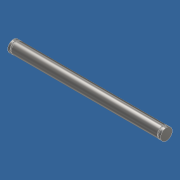
# Autodesk Inventor part: AxeHorizontalRoller
Saved by Autodesk Inventor 2018 (Build 220112000, 112)
## iProperties
Created: 2022-02-22
Part Number: AxeHorizontalRoller
Material: Stainless Steel
Document SubType Name: Modeling
Designer: Nathann
Density: 8 g/cm^3
Appearance: Semi-Polished
Mass: 40.2279 g
Surface Area: 30.1308 cm^2
Volume: 5.02849 cm^3
Author: Nathann
Autodesk Inventor part; units mm, degrees
ref_plane "YZ Plane" through (0, 0, 0) normal (1, 0, 0) x (0, 1, 0)
ref_plane "XZ Plane" through (0, 0, 0) normal (0, 1, 0) x (-1, 0, 0)
sketch "Sketch1" plane through (0, 0, 0) normal (1, 0, 0) x (0, 1, 0)
  arc A0 (-0.9778, 3.8786) -> (1.0222, 3.8672) centre (0, 0) ccw
  circle A1 centre (0, 0) radius 4
  dimension "d0" = 8
  constraints: 2 coincident, 2 point on circle, 1 centre point, 3 other
  measures "d0" diameter of A0
extrude "Extrusion1" add sketch "Sketch1" against normal blind 105
sketch "Sketch2" plane through (0, 0, 0) normal (0, 0, 1) x (1, 0, 0)
  line L0 (-2.44, 6.5) -> (-1.5, 6.5)
  line L1 (-1.5, 6.5) -> (-1.5, 3.5)
  line L2 (-1.5, 3.5) -> (-2.44, 3.5)
  line L3 (-2.44, 3.5) -> (-2.44, 6.5)
  line L4 (0, 4) -> (0, -4) projected
  line L5 (0, 4) -> (-105, 4) projected
  line L6 (-126, 0) -> (21, 0) projected
  line L7 (0, 4) -> (-105, 4) projected
  line L8 (-52.5, 4) -> (-52.5, -9.5088)
  line L9 (-102.56, 6.5) -> (-103.5, 6.5)
  line L10 (-103.5, 6.5) -> (-103.5, 3.5)
  line L11 (-103.5, 3.5) -> (-102.56, 3.5)
  line L12 (-102.56, 3.5) -> (-102.56, 6.5)
  line L13 (-105, 4) -> (-105, -4)
  line L14 (0, -4) -> (-105, -4) projected
  point P0 (0, 0)
  point P1 (0, 1.0222)
  point P2 (0, -0.9778)
  point P3 (-105, 0)
  point P4 (-105, 1.0222)
  point P5 (-105, -0.9778)
  dimension "d9" = 1.5
  dimension "d10" = 0.94
  dimension "d11" = 0.5
  dimension "d12" = 3
  dimension "d18" = 8
  constraints: 20 end point, 11 symmetric about line, 2 parallel, 1 horizontal, 1 midpoint, 1 perpendicular, 1 vertical
  measures "d9" distance between parallel lines of L4 L1
  measures "d10" distance of L1.end L2.end
  measures "d11" distance between parallel lines of L5 L2
  measures "d12" distance of L2.end L0.start
  measures "d18" distance between parallel lines of L5 L14
revolve "Revolution1" cut sketch "Sketch2" angle 360 about axis through (-10, 0, 0) along (1, 0, 0) contours L0 L1 L5 L3 | L5 L1 L2 L3 | L12 L11 L10 L5 | L5 L10 L9 L12
ref_plane "Work Plane1" through (0, 0, -4) normal (0, 0, 1) x (1, 0, 0)
sketch "Sketch5" plane through (0, 0, -4) normal (0, 0, 1) x (1, 0, 0)
  line L0 (-73, 1) -> (-55, 1)
  line L1 (-55, 1) -> (-55, -1)
  line L2 (-55, -1) -> (-73, -1)
  line L3 (-73, -1) -> (-73, 1)
  line L4 (-2.44, -4) -> (-102.56, -4) projected
  line L5 (-2.44, 4) -> (-102.56, 4) projected
  line L6 (-105, 4) -> (-105, -4) projected
  circle A0 centre (-55, 0) radius 1
  circle A1 centre (-73, 0) radius 1
  line L7 (-42.5, 1) -> (-24.5, 1)
  line L8 (-24.5, 1) -> (-24.5, -1)
  line L9 (-24.5, -1) -> (-42.5, -1)
  line L10 (-42.5, -1) -> (-42.5, 1)
  circle A2 centre (-24.5, 0) radius 1
  circle A3 centre (-42.5, 0) radius 1
  line L11 (0, 4) -> (0, -4) projected
  point P0 (0, 0)
  dimension "d24" = 20
  dimension "d19" = 2
  dimension "d20" = 8
  dimension "d21" = 3
  dimension "d22" = 32
  dimension "d23" = 18
  dimension "d25" = 2
  dimension "d26" = 24.5
  dimension "d27" = 18
  constraints: 16 end point, 4 midpoint, 4 parallel, 4 vertical alignment, 2 horizontal, 2 perpendicular, 8 other
  measures "d19" distance between parallel lines of L0 L2
  measures "d20" distance between parallel lines of L5 L4
  measures "d21" distance between parallel lines of L2 L4
  measures "d22" distance between parallel lines of L6 L3
  measures "d23" distance of point (-73, 0) point (-55, 0)
  measures "d25" distance between parallel lines of L7 L9
  measures "d26" distance from line of point (-24.5, 0) L11
  measures "d27" distance of point (-42.5, 0) point (-24.5, 0)
extrude "Extrusion4" cut sketch "Sketch5" along normal blind 1.2
equation "\"d21\" = 0.5 * d20 - 0.5 * d19"
equation "\"d27\" = d23"
body "Solid1"
